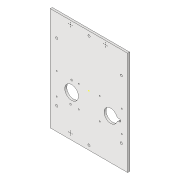
# Autodesk Inventor part: BREEZE-M10
Saved by Autodesk Inventor 2020 (Build 240168000, 168)
## iProperties
Created: 2020-04-12
Part Number: BREEZE-M10
Material: Generic
Description: TOP PANEL
Document SubType Name: Modeling
Designer: John K
Density: 1 g/cm^3
Appearance: Default
Author: John K
Autodesk Inventor part; units mm, degrees
ref_plane "YZ Plane" through (0, 0, 0) normal (1, 0, 0) x (0, 1, 0)
ref_plane "XZ Plane" through (0, 0, 0) normal (0, 1, 0) x (-1, 0, 0)
ref_plane "XY Plane" through (0, 0, 0) normal (0, 0, 1) x (1, 0, 0)
sketch "Face" plane through (0, 0, 0) normal (0, 0, 1) x (1, 0, 0)
  circle A0 centre (165.25, 188.4851) radius 2.6
  line L0 (158.2922, 98.7156) -> (160.7871, 98.7156)
  line L1 (160.7871, 92.4666) -> (158.965, 92.4666)
  arc A1 (158.965, 92.4666) -> (155.1773, 89.7524) centre (158.965, 88.4666) ccw
  circle A2 centre (114.75, 121.9851) radius 1.4
  arc A3 (154.6425, 101.0786) -> (155.1773, 89.7524) centre (140.5, 94.7351) ccw
  circle A4 centre (166.25, 70.4851) radius 1.4
  circle A5 centre (66.134, 121.9851) radius 1.4
  circle A6 centre (49.495, 121.2351) radius 2
  line L2 (180, 0) -> (180, 240.4851)
  line L3 (0, 0) -> (0, 240.4851)
  circle A7 centre (49.495, 96.2351) radius 16
  circle A8 centre (66.134, 70.4851) radius 1.4
  circle A9 centre (47.0211, 71.2351) radius 2
  line L4 (0, 0) -> (180, 0)
  circle A10 centre (90, 10) radius 2.6
  circle A11 centre (14.634, 121.9851) radius 1.4
  arc A12 (154.6425, 101.0786) -> (158.2922, 98.7156) centre (158.2922, 102.7156) ccw
  circle A13 centre (14.75, 52) radius 2.6
  circle A14 centre (90, 230.4851) radius 2.6
  circle A15 centre (14.75, 188.4851) radius 2.6
  circle A16 centre (165.25, 52) radius 2.6
  line L5 (180, 240.4851) -> (0, 240.4851)
  circle A17 centre (166.25, 121.9851) radius 1.4
  circle A18 centre (14.634, 70.4851) radius 1.4
  arc A19 (160.7871, 92.4666) -> (160.7871, 98.7156) centre (160.7871, 95.5911) ccw
  circle A20 centre (114.75, 70.4851) radius 1.4
  point P0 (106.7876, 102.9578)
sketch "Sketch1" plane through (0, 0, 0) normal (0, 0, 1) x (1, 0, 0)
  circle A0 centre (75.25, 68.2425) radius 2.6
  line L0 (68.2922, -21.527) -> (70.7871, -21.527)
  line L1 (70.7871, -27.776) -> (68.965, -27.776)
  arc A1 (68.965, -27.776) -> (65.1773, -30.4901) centre (68.965, -31.776) ccw
  circle A2 centre (24.75, 1.7425) radius 1.4
  arc A3 (64.6425, -19.164) -> (65.1773, -30.4901) centre (50.5, -25.5075) ccw
  circle A4 centre (76.25, -49.7575) radius 1.4
  circle A5 centre (-23.866, 1.7425) radius 1.4
  circle A6 centre (-40.505, 0.9925) radius 2
  line L2 (90, -120.2425) -> (90, 120.2425)
  line L3 (-90, -120.2425) -> (-90, 120.2425)
  circle A7 centre (-40.505, -24.0075) radius 16
  circle A8 centre (-23.866, -49.7575) radius 1.4
  circle A9 centre (-42.9789, -49.0075) radius 2
  line L4 (-90, -120.2425) -> (90, -120.2425)
  circle A10 centre (0, -110.2425) radius 2.6
  circle A11 centre (-75.366, 1.7425) radius 1.4
  arc A12 (64.6425, -19.164) -> (68.2922, -21.527) centre (68.2922, -17.527) ccw
  circle A13 centre (-75.25, -68.2425) radius 2.6
  circle A14 centre (0, 110.2425) radius 2.6
  circle A15 centre (-75.25, 68.2425) radius 2.6
  circle A16 centre (75.25, -68.2425) radius 2.6
  line L5 (90, 120.2425) -> (-90, 120.2425)
  circle A17 centre (76.25, 1.7425) radius 1.4
  circle A18 centre (-75.366, -49.7575) radius 1.4
  arc A19 (70.7871, -27.776) -> (70.7871, -21.527) centre (70.7871, -24.6515) ccw
  circle A20 centre (24.75, -49.7575) radius 1.4
  point P0 (0, 0)
  point P1 (90, 0)
  point P2 (0, -120.2425)
  constraints: 1 horizontal alignment, 1 vertical alignment, 2 other
extrude "Extrusion1" add sketch "Sketch1" along normal mid plane 4.75
sketch "Sketch2" plane through (0, 0, 2.375) normal (0, 0, 1) x (1, 0, 0)
  circle A0 centre (0, 110.2425) radius 2.6 projected
  circle A1 centre (0, -110.2425) radius 2.6 projected
  point P0 (0, 0)
  point P1 (46.8313, 110.2425)
  point P2 (-46.8312, 110.2425)
  point P3 (-46.8312, -110.2425)
  point P4 (46.8313, 110.2425)
  point P5 (46.8313, -110.2425)
  dimension "d2" = 93.6625
  dimension "d3" = 46.8312
  constraints: 4 horizontal alignment, 2 coincident, 2 vertical alignment
  measures "d2" distance of point (-46.831, 110.243) point (46.831, 110.243)
  measures "d3" distance of A0.centre point (46.831, 110.243)
hole "Hole1" at (46.8313, 110.2425, 2.375) at (-46.8312, 110.2425, 2.375) at (-46.8312, -110.2425, 2.375) at (46.8313, -110.2425, 2.375) direction (0, 0, -1) diameter 5.5 end through all clearance for "Socket Head Cap Screw" size "M5" standard "Ansi Metric M Profile"
equation "\"d3\" = 0.5 * d2"
body "Solid1"
